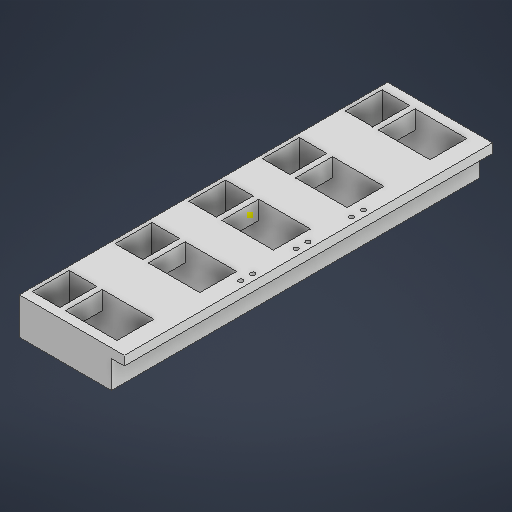
# Autodesk Inventor part: Fem_Sensor_Indtil_Videre
Saved by Autodesk Inventor 2026.1 (Build 301233020, 233B)
## iProperties
Created: 2025-10-29
Part Number: Fem_Sensor_Indtil_Videre
Material: Generic
Document SubType Name: Modeling
Designer: willi
Density: 1 g/cm^3
Appearance: Default
Author: willi
Autodesk Inventor part; units mm, degrees
ref_plane "YZ Plane" through (0, 0, 0) normal (1, 0, 0) x (0, 1, 0)
ref_plane "XZ Plane" through (0, 0, 0) normal (0, 1, 0) x (-1, 0, 0)
ref_plane "XY Plane" through (0, 0, 0) normal (0, 0, 1) x (1, 0, 0)
sketch "Sketch1" plane through (0, 0, 0) normal (0, 1, 0) x (-1, 0, 0)
  line L0 (-25, -100) -> (25, -100)
  line L1 (25, -100) -> (25, 100)
  line L2 (25, 100) -> (-25, 100)
  line L3 (-25, 100) -> (-25, -100)
  line L4 (-25, -100) -> (25, 100) construction
  line L5 (25, -100) -> (-25, 100) construction
  line L6 (23, 50) -> (-23, 50)
  line L7 (-23, 50) -> (-23, 30)
  line L8 (-23, 30) -> (23, 30)
  line L9 (23, 30) -> (23, 50)
  line L10 (23, 50) -> (-23, 30) construction
  line L11 (-23, 50) -> (23, 30) construction
  line L12 (23, -30) -> (-23, -30)
  line L13 (-23, -30) -> (-23, -50)
  line L14 (-23, -50) -> (23, -50)
  line L15 (23, -50) -> (23, -30)
  line L16 (23, -30) -> (-23, -50) construction
  line L17 (-23, -30) -> (23, -50) construction
  line L18 (-23, 10) -> (23, 10)
  line L19 (23, 10) -> (23, -10)
  line L20 (23, -10) -> (-23, -10)
  line L21 (-23, -10) -> (-23, 10)
  line L22 (-23, 10) -> (23, -10) construction
  line L23 (23, 10) -> (-23, -10) construction
  line L24 (-23, 95) -> (23, 95)
  line L25 (23, 95) -> (23, 75)
  line L26 (23, 75) -> (-23, 75)
  line L27 (-23, 75) -> (-23, 95)
  line L28 (-23, 95) -> (23, 75) construction
  line L29 (23, 95) -> (-23, 75) construction
  line L30 (-23, -75) -> (23, -75)
  line L31 (23, -75) -> (23, -95)
  line L32 (23, -95) -> (-23, -95)
  line L33 (-23, -95) -> (-23, -75)
  line L34 (-23, -75) -> (23, -95) construction
  line L35 (23, -75) -> (-23, -95) construction
  point P0 (0, 0)
  point P1 (0, 40)
  point P2 (0, -40)
  point P3 (0, 0)
  point P4 (0, 85)
  point P5 (0, -85)
  dimension "d0" = 200
  dimension "d1" = 50
  dimension "d2" = 2
  dimension "d3" = 46
  dimension "d4" = 20
  dimension "d5" = 46
  dimension "d6" = 20
  dimension "d7" = 2
  dimension "d8" = 20
  dimension "d9" = 46
  dimension "d10" = 2
  dimension "d11" = 0
  dimension "d12" = 20
  dimension "d13" = 20
  dimension "d14" = 46
  dimension "d15" = 20
  dimension "d16" = 20
  dimension "d17" = 46
  dimension "d18" = 2
  dimension "d19" = 2
  dimension "d20" = 25
  dimension "d21" = 25
  constraints: 72 end point, 12 midpoint, 12 parallel, 6 horizontal, 6 perpendicular
  measures "d0" distance of L0.end L1.end
  measures "d1" distance of L1.end L2.end
  measures "d2" distance between parallel lines of L3 L7
  measures "d3" distance of L7.end L8.end
  measures "d4" distance of L6.end L7.end
  measures "d5" distance of L19.end L20.end
  measures "d6" distance of L18.end L19.end
  measures "d7" distance between parallel lines of L3 L21
  measures "d8" distance of L12.end L13.end
  measures "d9" distance of L12.start L12.end
  measures "d10" distance between parallel lines of L3 L13
  measures "d11" distance of point (0, 0) point (0, 0)
  measures "d12" distance between parallel lines of L12 L20
  measures "d13" distance between parallel lines of L8 L18
  measures "d14" distance of L30.start L30.end
  measures "d15" distance of L32.end L30.start
  measures "d16" distance of L26.end L24.start
  measures "d17" distance of L25.end L26.end
  measures "d18" distance between parallel lines of L3 L27
  measures "d19" distance between parallel lines of L3 L33
  measures "d20" distance between parallel lines of L6 L26
  measures "d21" distance between parallel lines of L14 L30
extrude "Extrusion1" add sketch "Sketch1" along normal blind 35
sketch "Sketch2" plane through (0, 35, 0) normal (0, 1, 0) x (1, 0, 0)
  line L0 (23, -95) -> (-23, -95) projected
  line L1 (-23, -75) -> (23, -75) projected
  line L2 (-8, -95) -> (-5, -95)
  line L3 (-5, -95) -> (-5, -75)
  line L4 (-5, -75) -> (-8, -75)
  line L5 (-8, -75) -> (-8, -95)
  line L6 (-23, -30) -> (23, -30) projected
  line L7 (-8, -50.2373) -> (-5, -50.2373)
  line L8 (-5, -50.2373) -> (-5, -30)
  line L9 (-5, -30) -> (-8, -30)
  line L10 (-8, -30) -> (-8, -50.2373)
  line L11 (-8, -10.1346) -> (-5, -10.1346)
  line L12 (-5, -10.1346) -> (-5, 9.9167)
  line L13 (-5, 9.9167) -> (-8, 9.9167)
  line L14 (-8, 9.9167) -> (-8, -10.1346)
  line L15 (-23, 50) -> (23, 50) projected
  line L16 (-8, 29.7501) -> (-5, 29.7501)
  line L17 (-5, 29.7501) -> (-5, 50)
  line L18 (-5, 50) -> (-8, 50)
  line L19 (-8, 50) -> (-8, 29.7501)
  line L20 (23, 75) -> (-23, 75) projected
  line L21 (-23, 95) -> (23, 95) projected
  line L22 (-8, 75) -> (-5, 75)
  line L23 (-5, 75) -> (-5, 95)
  line L24 (-5, 95) -> (-8, 95)
  line L25 (-8, 95) -> (-8, 75)
  line L26 (-23, -95) -> (-23, -75) projected
  line L27 (-23, 75) -> (-23, 95) projected
  point P0 (0, 0)
  dimension "d24" = 3
  dimension "d25" = 3
  dimension "d26" = 3
  dimension "d27" = 3
  dimension "d28" = 3
  dimension "d29" = 15
  dimension "d30" = 15
  constraints: 40 end point, 10 parallel, 9 point on line, 5 horizontal, 5 perpendicular
  measures "d24" distance between parallel lines of L3 L5
  measures "d25" distance between parallel lines of L8 L10
  measures "d26" distance between parallel lines of L12 L14
  measures "d27" distance between parallel lines of L17 L19
  measures "d28" distance between parallel lines of L23 L25
  measures "d29" distance between parallel lines of L26 L5
  measures "d30" distance between parallel lines of L27 L25
extrude "Extrusion2" add sketch "Sketch2" against normal blind 10 contours L0 L5 L1 L3 | L6 L8 L7 L10 | L14 L13 L12 L11 | L15 L17 L16 L19 | L20 L25 L21 L23
sketch "Sketch3" plane through (0, 35, 0) normal (0, 1, 0) x (1, 0, 0)
  line L0 (-5, -10) -> (-5, 9.9167) projected
  line L1 (-8, 30) -> (-8, 50) projected
  line L2 (-5, 8.437) -> (-8, 8.437)
  line L3 (-8, 8.437) -> (-8, 32.4131)
  line L4 (-8, 32.4131) -> (-5, 32.4131)
  line L5 (-5, 32.4131) -> (-5, 8.437)
  point P0 (0, 0)
  constraints: 8 end point, 2 parallel, 2 point on line, 1 horizontal, 1 perpendicular
extrude "Extrusion3" add sketch "Sketch3" against normal blind 10
sketch "Sketch4" plane through (25, 0, -100) normal (0, 0, -1) x (-1, 0, 0)
  line L0 (0, 35) -> (-7, 35)
  line L1 (-7, 35) -> (-7, 30)
  line L2 (-7, 30) -> (0, 30)
  line L3 (0, 30) -> (0, 35)
  line L4 (0, 0) -> (0, 35) projected
  line L5 (0, 35) -> (50, 35) projected
  point P0 (25, 0)
  dimension "d35" = 0
  dimension "d36" = 7
  dimension "d37" = 5
  dimension "d38" = 0
  constraints: 8 end point, 2 parallel, 1 horizontal, 1 perpendicular
  measures "d35" distance between parallel lines of L4 L3
  measures "d36" distance of L1.end L2.end
  measures "d37" distance of L0.end L1.end
  measures "d38" distance between parallel lines of L5 L0
extrude "Extrusion4" add sketch "Sketch4" against normal blind 200
sketch "Sketch5" plane through (25, 0, -100) normal (0, 0, -1) x (-1, 0, 0)
  point P0 (25, 0)
sketch "Sketch6" plane through (0, 35, 0) normal (0, 1, 0) x (1, 0, 0)
  circle A0 centre (28.5, -33.25) radius 1.25
  circle A1 centre (28.5, -26.75) radius 1.25
  line L0 (32, 100) -> (32, -100)
  circle A2 centre (28.5, -3.25) radius 1.25
  circle A3 centre (28.5, 3.25) radius 1.25
  circle A4 centre (28.5, 26.75) radius 1.25
  circle A5 centre (28.5, 33.25) radius 1.25
  line L1 (-25, 100) -> (32, 100)
  line L2 (-25, -100) -> (32, -100)
  point P0 (0, 0)
  dimension "d41" = 2.5
  dimension "d42" = 2.5
  dimension "d46" = 2.5
  dimension "d47" = 2.5
  dimension "d48" = 2.5
  dimension "d49" = 2.5
  dimension "d51" = 4
  dimension "d53" = 4
  dimension "d54" = 3.5
  dimension "d55" = 3.5
  dimension "d56" = 3.5
  dimension "d57" = 4
  dimension "d58" = 3.5
  dimension "d59" = 3.5
  dimension "d62" = 96.75
  dimension "d63" = 3.5
  dimension "d66" = 21
  dimension "d67" = 21
  constraints: 6 centre point, 6 end point
  measures "d41" diameter of A0
  measures "d42" diameter of A1
  measures "d46" diameter of A4
  measures "d47" diameter of A5
  measures "d48" diameter of A3
  measures "d49" diameter of A2
  measures "d54" distance from line of L0 A0.centre
  measures "d55" distance from line of L0 A4.centre
  measures "d56" distance from line of L0 A5.centre
  measures "d58" distance from line of L0 A3.centre
  measures "d59" distance from line of L0 A2.centre
  measures "d62" distance from line of L2 A2.centre
  measures "d63" distance from line of L0 A1.centre
extrude "Extrusion5" cut sketch "Sketch6" against normal blind 30
sketch "Sketch7" plane through (25, 0, -100) normal (0, 0, -1) x (-1, 0, 0)
  point P0 (25, 0)
sketch "Sketch8" plane through (0, 35, 0) normal (0, 1, 0) x (1, 0, 0)
  point P0 (0, 0)
sketch "Sketch9" plane through (25, 0, 100) normal (1, 0, 0) x (0, 0, -1)
  line L0 (-3.3992, 0) -> (201.6008, 0)
  line L1 (201.6008, 0) -> (201.6008, 15)
  line L2 (201.6008, 15) -> (-3.3992, 15)
  line L3 (-3.3992, 15) -> (-3.3992, 0)
  line L4 (0, 0) -> (200, 0) projected
  point P0 (100, 0)
  dimension "d68" = 15
  dimension "d69" = 0
  dimension "d70" = 205
  constraints: 8 end point, 2 parallel, 1 horizontal, 1 perpendicular
  measures "d68" distance of L2.end L0.start
  measures "d69" distance between parallel lines of L4 L0
  measures "d70" distance of L1.end L2.end
extrude "Extrusion6" cut sketch "Sketch9" against normal blind 55
body "Solid1"
